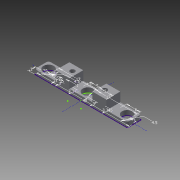
# Autodesk Inventor part: Bar_Extruded
Saved by Autodesk Inventor 2014 SP1 (Build 180222100, 222)
## iProperties
Created: 2015-03-26
Part Number: Bar_Extruded
Material: Generic
Document SubType Name: Modeling
Designer: Erin
Density: 1 g/cm^3
Appearance: Default
Author: Erin
Autodesk Inventor part; units mm, degrees
ref_plane "YZ Plane" through (0, 0, 0) normal (1, 0, 0) x (0, 1, 0)
ref_plane "XZ Plane" through (0, 0, 0) normal (0, 1, 0) x (-1, 0, 0)
ref_plane "XY Plane" through (0, 0, 0) normal (0, 0, 1) x (1, 0, 0)
sketch "Sketch1" plane through (0, 0, 0) normal (0, 0, 1) x (1, 0, 0)
  line L0 (-20, -3) -> (20, -3) construction
  circle A0 centre (-17, 0) radius 2.25
  circle A1 centre (17, 0) radius 2.25
  circle A2 centre (0, 0) radius 2.25
  circle A3 centre (-7, 0.3446) radius 1
  circle A4 centre (7, 0.3446) radius 1
  line L1 (-23.9554, 0) -> (25.6733, 0) construction
  line L2 (0, 11.421) -> (0, -11.2937) construction
  line L3 (-20, -3) -> (20, -3)
  line L4 (20, -3) -> (20, 3)
  line L5 (20, 3) -> (-20, 3)
  line L6 (-20, 3) -> (-20, -3)
  circle A5 centre (-11.8345, 1.6861) radius 0.5
  line L7 (-11, 3) -> (-5, 3)
  line L8 (-5, 3) -> (-5, -3)
  line L9 (-5, -3) -> (-11, -3)
  line L10 (-11, -3) -> (-11, 3)
  line L11 (5, 3) -> (11, 3)
  line L12 (11, 3) -> (11, -3)
  line L13 (11, -3) -> (5, -3)
  line L14 (5, -3) -> (5, 3)
  point P0 (0, 0)
  point P1 (0, -3)
  point P2 (0, -3)
  point P3 (-2.8751, -5.808)
  point P4 (2.8751, -5.808)
  dimension "d0" = 40
  dimension "d1" = 4.5
  dimension "d2" = 4.5
  dimension "d3" = 3
  dimension "d4" = 4.5
  dimension "d5" = 3
  dimension "d6" = 3.3446
  dimension "d7" = 3.3446
  dimension "d8" = 3
  dimension "d9" = 17
  dimension "d10" = 17
  dimension "d11" = 3
  dimension "d12" = 3
  dimension "d13" = 3
  dimension "d14" = 3
  dimension "d16" = 1
  dimension "d20" = 6
  dimension "d22" = 5
  dimension "d23" = 5
  dimension "d24" = 6
  constraints: 30 end point, 7 parallel, 6 centre point, 6 point on line, 4 horizontal, 4 perpendicular, 1 coincident, 1 midpoint, 1 vertical
  measures "d0" distance of L0.start L0.end
  measures "d1" diameter of A0
  measures "d2" diameter of A1
  measures "d3" distance from line of A0.centre L0
  measures "d4" diameter of A2
  measures "d5" distance from line of A2.centre L0
  measures "d6" distance from line of A3.centre L0
  measures "d7" distance from line of A4.centre L0
  measures "d8" distance between parallel lines of L0 L1
  measures "d9" distance from line of L2 A1.centre
  measures "d10" distance from line of L2 A0.centre
  measures "d11" distance from line of A0.centre L3
  measures "d12" distance from line of A0.centre L6
  measures "d13" distance from line of A0.centre L5
  measures "d14" distance from line of A1.centre L4
  measures "d16" diameter of A5
  measures "d20" distance from line of A0.centre L10
  measures "d22" distance between parallel lines of L2 L8
  measures "d23" distance between parallel lines of L2 L14
  measures "d24" distance from line of A1.centre L12
extrude "Extrusion1" add sketch "Sketch1" along normal blind 2
fillet "Fillet1" radius 1 4 edges at (-20, 3, 1) (-20, -3, 1) (20, 3, 1) (20, -3, 1)
extrude "Extrusion2" add sketch "Sketch1" along normal blind 6 contours L10 L5 L8 L3 | L14 L5 L12 L3
body "Solid1"
